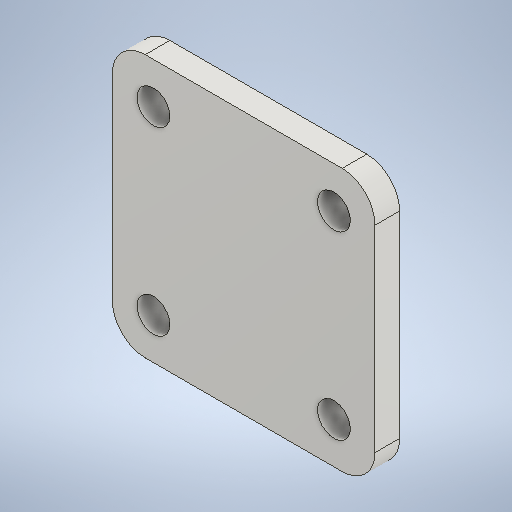
# Autodesk Inventor part: 12A VALVE BONNET
Saved by Autodesk Inventor 2025.2 (Build 292293000, 293)
## iProperties
Created: 2025-05-29
Part Number: 12A VALVE BONNET
Material: Steel AISI 1020 107 HR
Document SubType Name: Modeling
Designer: bless
Density: 7.87 g/cm^3
Appearance: Steel
Author: bless
Autodesk Inventor part; units mm, degrees
ref_plane "YZ Plane" through (0, 0, 0) normal (1, 0, 0) x (0, 1, 0)
ref_plane "XZ Plane" through (0, 0, 0) normal (0, 1, 0) x (-1, 0, 0)
ref_plane "XY Plane" through (0, 0, 0) normal (0, 0, 1) x (1, 0, 0)
sketch "Sketch1" plane through (0, 0, 0) normal (0, 0, 1) x (1, 0, 0)
  line L0 (-6, 8) -> (6, 8)
  line L1 (8, 6) -> (8, -6)
  line L2 (6, -8) -> (-6, -8)
  line L3 (-8, -6) -> (-8, 6)
  line L4 (-8, 8) -> (8, -8) construction
  line L5 (8, 8) -> (-8, -8) construction
  arc A0 (-6, 8) -> (-8, 6) centre (-6, 6) ccw
  arc A1 (-8, -6) -> (-6, -8) centre (-6, -6) ccw
  arc A2 (6, -8) -> (8, -6) centre (6, -6) ccw
  arc A3 (8, 6) -> (6, 8) centre (6, 6) ccw
  point P0 (0, 0)
  dimension "d0" = 16
  dimension "d1" = 16
  dimension "d2" = 2
  constraints: 12 end point, 8 point on circle, 8 point on line, 8 tangent, 4 centre point, 3 equal radius, 2 midpoint, 2 parallel, 1 horizontal, 1 perpendicular
  measures "d0" distance of L4.start L5.start
  measures "d1" distance between parallel lines of L2 L0
  measures "d2" radius of A0
extrude "Extrusion1" add sketch "Sketch1" along normal blind 1.5
sketch "Sketch2" plane through (0, 0, 1.5) normal (0, 0, 1) x (1, 0, 0)
  line L0 (-6, -8) -> (6, -8) projected
  line L1 (8, -6) -> (8, 6) projected
  line L2 (6, 8) -> (-6, 8) projected
  line L3 (-8, 6) -> (-8, -6) projected
  circle A0 centre (-5.5, 5.5) radius 1
  circle A1 centre (5.5, 5.5) radius 1
  circle A2 centre (5.5, -5.5) radius 1
  circle A3 centre (-5.5, -5.5) radius 1
  point P0 (0, 0)
  dimension "d5" = 2
  dimension "d6" = 2.5
  dimension "d7" = 2.5
  dimension "d8" = 2.5
  dimension "d9" = 2.5
  constraints: 4 centre point, 3 equal radius, 2 horizontal alignment, 2 vertical alignment
  measures "d5" diameter of A0
  measures "d6" distance from line of L2 A0.centre
  measures "d7" distance from line of L3 A0.centre
  measures "d8" distance from line of L1 A1.centre
  measures "d9" distance from line of L0 A3.centre
extrude "Extrusion2" cut sketch "Sketch2" against normal through all
body "Solid1"
